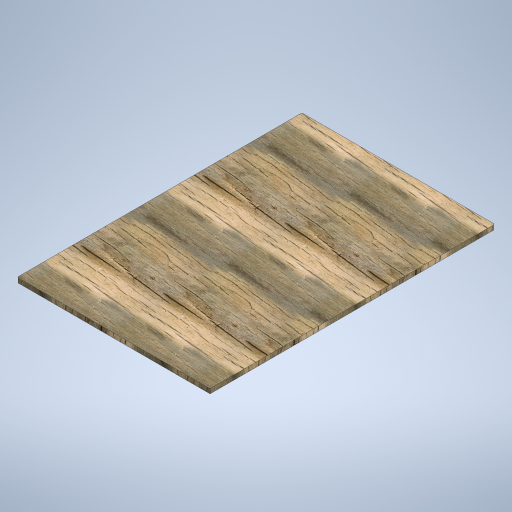
# Autodesk Inventor part: Tutup_Box
Saved by Autodesk Inventor 2023.1 (Build 271208000, 208)
## iProperties
Created: 2024-03-27
Part Number: Tutup_Box
Material: Generic
Document SubType Name: Modeling
Designer: bahariridwan
Density: 1 g/cm^3
Appearance: Driftwood
Author: bahariridwan
Autodesk Inventor part; units mm, degrees
ref_plane "YZ Plane" through (0, 0, 0) normal (1, 0, 0) x (0, 1, 0)
ref_plane "XZ Plane" through (0, 0, 0) normal (0, 1, 0) x (-1, 0, 0)
ref_plane "XY Plane" through (0, 0, 0) normal (0, 0, 1) x (1, 0, 0)
sketch "Sketch1" plane through (0, 0, 0) normal (0, 1, 0) x (-1, 0, 0)
  line L0 (0, 0) -> (210, 0)
  line L1 (210, 0) -> (210, -310)
  line L2 (210, -310) -> (0, -310)
  line L3 (0, -310) -> (0, 0)
  dimension "d0" = 310
  dimension "d1" = 210
  constraints: 8 end point, 2 parallel, 1 horizontal, 1 perpendicular
  measures "d0" distance of L0.end L1.end
  measures "d1" distance of L1.end L2.end
extrude "Extrusion1" add sketch "Sketch1" along normal blind 5
chamfer "Chamfer1" distance 1 angle 45 4 edges at (0, 2.5, -310) (0, 2.5, 0) (-210, 2.5, -310) (-210, 2.5, 0)
sketch "Sketch2" plane through (0, 0, 0) normal (0, -1, 0) x (1, 0, 0)
  line L0 (-205, -305) -> (-5, -305)
  line L1 (-5, -305) -> (-5, -5)
  line L2 (-5, -5) -> (-205, -5)
  line L3 (-205, -5) -> (-205, -305)
  line L4 (0, -1) -> (0, -309) projected
  line L5 (-209, 0) -> (-1, 0) projected
  point P0 (0, 0)
  dimension "d7" = 300
  dimension "d8" = 200
  dimension "d9" = 5
  dimension "d10" = 5
  constraints: 8 end point, 2 parallel, 1 horizontal, 1 perpendicular
  measures "d7" distance of L2.end L0.start
  measures "d8" distance of L1.end L2.end
  measures "d9" distance between parallel lines of L4 L1
  measures "d10" distance between parallel lines of L5 L2
extrude "Extrusion2" add sketch "Sketch2" along normal blind 5
sketch "Sketch3" plane through (0, -5, 0) normal (0, -1, 0) x (1, 0, 0)
  line L0 (-195, -295) -> (-15, -295)
  line L1 (-15, -295) -> (-15, -15)
  line L2 (-15, -15) -> (-195, -15)
  line L3 (-195, -15) -> (-195, -295)
  line L4 (-5, -5) -> (-205, -5) projected
  line L5 (-205, -5) -> (-205, -305) projected
  point P0 (0, 0)
  dimension "d13" = 280
  dimension "d14" = 180
  dimension "d15" = 10
  dimension "d16" = 10
  constraints: 8 end point, 2 parallel, 1 horizontal, 1 perpendicular
  measures "d13" distance of L2.end L0.start
  measures "d14" distance of L1.end L2.end
  measures "d15" distance between parallel lines of L4 L2
  measures "d16" distance between parallel lines of L5 L3
extrude "Extrusion3" cut sketch "Sketch3" against normal blind 5
body "Solid1"
